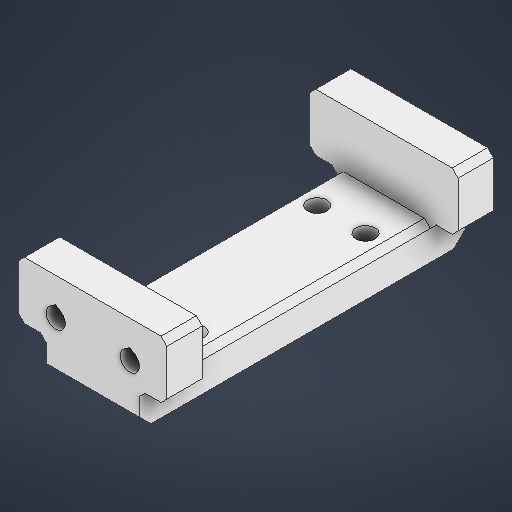
# Autodesk Inventor part: CNC-023-YAxisBallScrewStabilizerMount
Saved by Autodesk Inventor 2026.2 (Build 302298000, 298)
## iProperties
Created: 2026-06-24
Part Number: CNC-023-YAxisBallScrewStabilizerMount
Material: ABS Plastic
Document SubType Name: Modeling
Designer: Kenji
Density: 1.06 g/cm^3
Appearance: Smooth - White
Author: Kenji
Autodesk Inventor part; units mm, degrees
ref_plane "YZ Plane" through (0, 0, 0) normal (1, 0, 0) x (0, 1, 0)
ref_plane "XZ Plane" through (0, 0, 0) normal (0, 1, 0) x (-1, 0, 0)
sketch "Sketch1" plane through (0, 0, 0) normal (0, 1, 0) x (-1, 0, 0)
  line L0 (-12.5, -44) -> (12.5, -44)
  line L1 (12.5, -44) -> (12.5, 44)
  line L2 (12.5, 44) -> (-12.5, 44)
  line L3 (-12.5, 44) -> (-12.5, -44)
  line L4 (-12.5, -44) -> (12.5, 44) construction
  line L5 (12.5, -44) -> (-12.5, 44) construction
  point P0 (0, 0)
  dimension "d0" = 88
  dimension "d1" = 25
  constraints: 12 end point, 2 midpoint, 2 parallel, 1 horizontal, 1 perpendicular
  measures "d0" distance between parallel lines of L0 L2
  measures "d1" distance of L0.start L0.end
extrude "Extrusion1" add sketch "Sketch1" along normal blind 9.525
sketch "Sketch2" plane through (0, 9.525, 0) normal (0, 1, 0) x (1, 0, 0)
  line L0 (20, -34.475) -> (-20, -34.475)
  line L1 (-20, -34.475) -> (-20, -44)
  line L2 (-20, -44) -> (20, -44)
  line L3 (20, -44) -> (20, -34.475)
  line L4 (20, -34.475) -> (-20, -44) construction
  line L5 (-20, -34.475) -> (20, -44) construction
  line L6 (-12.5, -44) -> (12.5, -44) projected
  point P0 (0, 0)
  point P1 (0, -39.2375)
  dimension "d4" = 40
  dimension "d5" = 9.525
  constraints: 12 end point, 2 midpoint, 2 parallel, 1 collinear, 1 horizontal, 1 perpendicular, 1 vertical alignment
  measures "d4" distance between parallel lines of L3 L1
  measures "d5" distance between parallel lines of L2 L0
extrude "Extrusion2" add sketch "Sketch2" along normal blind 15.475
fillet "Fillet1" radius 3.175 6 edges at (-12.5, 9.525, 39.2375) (-20, 9.525, 39.2375) (-20, 25, 39.2375) (20, 9.525, 39.2375) (20, 25, 39.2375) (12.5, 9.525, 39.2375)
ref_plane "Work Plane1" through (-16.825, 25, 0) normal (0, 0, 1) x (1, 0, 0)
mirror "Mirror1" about plane through (-16.825, 25, 0) normal (0, 0, 1) of "Extrusion2", "Fillet1"
sketch "Sketch3" plane through (16.825, 25, -44) normal (0, 0, -1) x (-1, 0, 0)
  line L0 (29.325, -25) -> (29.325, -18.65) projected
  arc A0 (32.5, -15.475) -> (29.325, -18.65) centre (32.5, -18.65) ccw projected
  line L1 (33.65, -15.475) -> (32.5, -15.475) projected
  arc A1 (33.65, -15.475) -> (36.825, -12.3) centre (33.65, -12.3) ccw projected
  line L2 (36.825, -12.3) -> (36.825, -3.175) projected
  arc A2 (36.825, -3.175) -> (33.65, 0) centre (33.65, -3.175) ccw projected
  line L3 (33.65, 0) -> (0, 0) projected
  arc A3 (0, 0) -> (-3.175, -3.175) centre (0, -3.175) ccw projected
  line L4 (-3.175, -12.3) -> (-3.175, -3.175) projected
  arc A4 (-3.175, -12.3) -> (0, -15.475) centre (0, -12.3) ccw projected
  line L5 (1.15, -15.475) -> (0, -15.475) projected
  arc A5 (4.325, -18.65) -> (1.15, -15.475) centre (1.15, -18.65) ccw projected
  line L6 (4.325, -25) -> (4.325, -18.65) projected
  circle A6 centre (26.825, -10) radius 2.6
  circle A7 centre (6.825, -10) radius 2.6
  line L7 (4.325, -25) -> (29.325, -25) projected
  point P0 (16.825, -25)
  dimension "d10" = 5.2
  dimension "d11" = 10
  dimension "d12" = 10
  dimension "d13" = 10
  constraints: 2 centre point, 1 equal radius, 1 horizontal alignment
  measures "d10" diameter of A6
  measures "d11" distance from line of L3 A6.centre
  measures "d12" distance from line of A6.centre L2
  measures "d13" distance from line of L4 A7.centre
extrude "Extrusion3" cut sketch "Sketch3" against normal through all contours A6 | A7
sketch "Sketch4" plane through (0, 0, 0) normal (0, -1, 0) x (1, 0, 0)
  line L0 (-6.5, -23) -> (6.5, -23) construction
  line L1 (6.5, -23) -> (6.5, 23) construction
  line L2 (6.5, 23) -> (-6.5, 23) construction
  line L3 (-6.5, 23) -> (-6.5, -23) construction
  line L4 (-6.5, -23) -> (6.5, 23) construction
  line L5 (6.5, -23) -> (-6.5, 23) construction
  circle A0 centre (6.5, 23) radius 2.6
  circle A1 centre (6.5, -23) radius 2.6
  circle A2 centre (-6.5, -23) radius 2.6
  circle A3 centre (-6.5, 23) radius 2.6
  point P0 (0, 0)
  dimension "d16" = 5.2
  dimension "d17" = 46
  dimension "d18" = 13
  constraints: 12 end point, 4 centre point, 4 coincident, 3 equal radius, 2 midpoint, 2 parallel, 1 horizontal, 1 perpendicular
  measures "d16" diameter of A0
  measures "d17" distance of L0.end L1.end
  measures "d18" distance of L2.end L1.end
extrude "Extrusion4" cut sketch "Sketch4" against normal through all
sketch "Sketch5" plane through (16.825, 25, -44) normal (0, 0, -1) x (-1, 0, 0)
  circle A0 centre (6.825, -10) radius 2.6 projected
  circle A1 centre (26.825, -10) radius 2.6 projected
  line L0 (5.3878, -7.8333) -> (6.825, -6.88)
  line L1 (6.825, -6.88) -> (8.2622, -7.8333)
  line L2 (25.3878, -7.8333) -> (26.825, -6.88)
  line L3 (26.825, -6.88) -> (28.2622, -7.8333)
  point P0 (16.825, -25)
  point P1 (6.825, -7.4)
  point P2 (26.825, -7.4)
  dimension "d21" = 0.52
  dimension "d22" = 5.2
  dimension "d23" = 0.52
  constraints: 8 end point, 6 point on circle, 4 tangent, 4 vertical alignment
  measures "d21" distance of point (6.825, -7.4) L0.end
  measures "d22" diameter of A0
  measures "d23" distance of L2.end point (26.825, -7.4)
extrude "Extrusion5" cut sketch "Sketch5" against normal through all contours A0 L0 L1 | A1 L2 L3
sketch "Sketch6" plane through (0, 9.525, 0) normal (0, 1, 0) x (1, 0, 0)
  circle A0 centre (-6.5, 23) radius 2.6 projected
  circle A1 centre (6.5, 23) radius 2.6 projected
  circle A2 centre (-6.5, -23) radius 2.6 projected
  circle A3 centre (6.5, -23) radius 2.6 projected
  circle A4 centre (-6.5, 23) radius 5
  circle A5 centre (6.5, 23) radius 5
  circle A6 centre (-6.5, -23) radius 5
  circle A7 centre (6.5, -23) radius 5
  point P0 (0, 0)
  dimension "d26" = 10
  constraints: 4 centre point, 4 coincident, 3 equal radius
  measures "d26" diameter of A4
extrude "Extrusion6" add sketch "Sketch6" against normal up to surface (9.525 mm away)
chamfer "Chamfer1" distance 3.175 angle 45 2 edges at (0, 0, -44) (0, 0, 44)
sketch "Sketch7" plane through (-16.825, 25, 44) normal (0, 0, 1) x (1, 0, 0)
  line L0 (29.325, -21.825) -> (4.325, -21.825) projected
  line L1 (29.325, -21.825) -> (29.325, -18.65) projected
  arc A0 (32.5, -15.475) -> (29.325, -18.65) centre (32.5, -18.65) ccw projected
  line L2 (32.5, -15.475) -> (33.65, -15.475) projected
  arc A1 (33.65, -15.475) -> (36.825, -12.3) centre (33.65, -12.3) ccw projected
  line L3 (36.825, -12.3) -> (36.825, -3.175) projected
  arc A2 (36.825, -3.175) -> (33.65, 0) centre (33.65, -3.175) ccw projected
  line L4 (0, 0) -> (33.65, 0) projected
  arc A3 (0, 0) -> (-3.175, -3.175) centre (0, -3.175) ccw projected
  line L5 (-3.175, -12.3) -> (-3.175, -3.175) projected
  arc A4 (-3.175, -12.3) -> (0, -15.475) centre (0, -12.3) ccw projected
  line L6 (0, -15.475) -> (1.15, -15.475) projected
  arc A5 (4.325, -18.65) -> (1.15, -15.475) centre (1.15, -18.65) ccw projected
  line L7 (4.325, -21.825) -> (4.325, -18.65) projected
  line L8 (5.3878, -7.8333) -> (6.825, -6.88) projected
  line L9 (6.825, -6.88) -> (8.2622, -7.8333) projected
  arc A6 (5.3878, -7.8333) -> (8.2622, -7.8333) centre (6.825, -10) ccw projected
  line L10 (25.3878, -7.8333) -> (26.825, -6.88) projected
  line L11 (26.825, -6.88) -> (28.2622, -7.8333) projected
  arc A7 (25.3878, -7.8333) -> (28.2622, -7.8333) centre (26.825, -10) ccw projected
  line L12 (-3.175, 0) -> (36.825, 0)
  line L13 (36.825, 0) -> (36.825, -15.475)
  line L14 (36.825, -15.475) -> (-3.175, -15.475)
  line L15 (-3.175, -15.475) -> (-3.175, 0)
  line L16 (0, 0) -> (33.65, 0) projected
  line L17 (36.825, -12.3) -> (36.825, -3.175) projected
  line L18 (32.5, -15.475) -> (33.65, -15.475) projected
  line L19 (-3.175, -12.3) -> (-3.175, -3.175) projected
  line L20 (29.325, -18.65) -> (29.325, -15.475)
  line L21 (4.325, -18.65) -> (4.325, -15.475)
  point P0 (16.825, -25)
  point P1 (0, -15.475)
  constraints: 12 end point, 4 collinear, 2 parallel, 2 perpendicular, 2 point on line, 1 horizontal, 1 tangent, 1 vertical
extrude "Extrusion7" add sketch "Sketch7" against normal up to surface (9.525 mm away) contours A1 L13 L14 | L14 L15 A4 | A2 L12 L13 | L15 L12 A3
extrude "Extrusion8" cut sketch "Sketch7" against normal through all contours L20 L14 A0 | A5 L14 L21
sketch "Sketch8" plane through (20, 25, 34.475) normal (0, 0, -1) x (-1, 0, 0)
  line L0 (7.5, -15.475) -> (7.5, -18.65) projected
  arc A0 (10.675, -15.475) -> (7.5, -18.65) centre (10.675, -18.65) ccw projected
  line L1 (29.325, -15.475) -> (10.675, -15.475) projected
  arc A1 (32.5, -18.65) -> (29.325, -15.475) centre (29.325, -18.65) ccw projected
  line L2 (32.5, -18.65) -> (32.5, -15.475) projected
  line L3 (40, -15.475) -> (32.5, -15.475) projected
  line L4 (40, 0) -> (40, -15.475) projected
  line L5 (0, 0) -> (40, 0) projected
  line L6 (0, -15.475) -> (0, 0) projected
  line L7 (0, -15.475) -> (7.5, -15.475) projected
  line L8 (8.5628, -7.8333) -> (10, -6.88) projected
  line L9 (10, -6.88) -> (11.4372, -7.8333) projected
  arc A2 (8.5628, -7.8333) -> (11.4372, -7.8333) centre (10, -10) ccw projected
  line L10 (28.5628, -7.8333) -> (30, -6.88) projected
  line L11 (30, -6.88) -> (31.4372, -7.8333) projected
  arc A3 (28.5628, -7.8333) -> (31.4372, -7.8333) centre (30, -10) ccw projected
  line L12 (7.5, -15.475) -> (32.5, -15.475)
  point P0 (20, -25)
  point P1 (10.675, -15.475)
  constraints: 2 end point, 1 collinear
extrude "Extrusion9" add sketch "Sketch8" along normal up to surface (68.95 mm away) contours L12 A0 L0 | L12 L2 A1
mirror "Mirror2" about plane through (-16.825, 25, 0) normal (0, 0, 1) of "Extrusion2"
chamfer "Chamfer2" distance 1.5875 angle 45 14 edges at (20, 25, 39.2375) (20, 9.525, 39.2375) (-20, 25, 39.2375) (-20, 9.525, 39.2375) (-12.5, 9.525, 39.2375) (-12.5, 9.525, -39.2375) (-20, 9.525, -39.2375) (-20, 25, -39.2375) (12.5, 9.525, -39.2375) (12.5, 9.525, 39.2375) (20, 25, -39.2375) (20, 9.525, -39.2375) (-12.5, 9.525, 0) (12.5, 9.525, 0)
equation "\"d12\" = d11"
equation "\"d13\" = d12"
equation "\"d21\" = 0.1 * d22"
equation "\"d23\" = d21"
body "Solid1"
